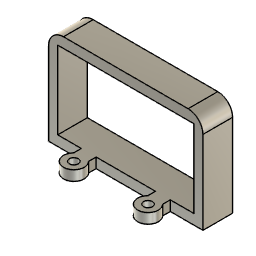
bat checker v5 (Autodesk Fusion 360 design; units mm, degrees)
Autodesk Fusion 360 part; units mm, degrees
note: some values were not read from the file. Set by a fixed rule: which sketch regions a step uses.
sketch "Sketch1" plane through (0, 0, 0) normal (0, 0, 1) x (1, 0, 0)
  line L0 (-65, 40) -> (-15, 40)
  line L1 (-15, 40) -> (-15, 50)
  line L2 (-15, 50) -> (-65, 50)
  line L3 (-65, 50) -> (-65, 40)
  dimension "d15" = 50
  constraint horizontal L0
  constraint vertical L1
  constraint horizontal L2
  constraint vertical L3
  measures "d15" distance of L0.start L0.end
extrude "Extrude4" add sketch "Sketch1" along normal blind 3
sketch "Sketch5" plane through (0, 0, 0) normal (0, 0, -1) x (1, 0, 0)
  line L0 (-65, -40) -> (-65, -50)
  line L1 (-65, -50) -> (-15, -50)
  line L2 (-15, -50) -> (-15, -40)
  line L3 (-15, -40) -> (-65, -40)
  line L4 (-65, -45) -> (-15, -45)
  line L5 (-15, -45) -> (-15, -50)
  line L6 (-15, -50) -> (-65, -50)
  line L7 (-65, -50) -> (-65, -45)
  constraint horizontal L4
  constraint vertical L5
  constraint horizontal L6
  constraint vertical L7
  constraint coincident L1.end L2.start
  constraint midpoint L0 L4.start
extrude "Extrude5" add sketch "Sketch5" along normal blind 30 contours L0 L1 L2 L4 L5 L6 L7
sketch "Sketch6" plane through (0, 50, 0) normal (0, 1, 0) x (-1, 0, 0)
  line L0 (65, -30) -> (65, 3)
  line L1 (65, 3) -> (15, 3)
  line L2 (15, 3) -> (15, -30)
  line L3 (15, -30) -> (65, -30)
  line L4 (17.55, -0.4) -> (62.45, -0.4)
  line L5 (62.45, -0.4) -> (62.45, -26.6)
  line L6 (62.45, -26.6) -> (17.55, -26.6)
  line L7 (17.55, -26.6) -> (17.55, -0.4)
  line L8 (17.55, -0.4) -> (62.45, -26.6) construction
  line L9 (62.45, -0.4) -> (17.55, -26.6) construction
  point P0 (40, -13.5)
  dimension "d24" = 44.9
  dimension "d25" = 26.2
  constraint horizontal L4
  constraint perpendicular L4 L5
  constraint parallel L4 L6
  constraint parallel L5 L7
  constraint coincident L8 P0
  constraint coincident L9 P0
  measures "d24" distance of L5.end L6.end
  measures "d25" distance of L4.end L5.end
extrude "Extrude6" cut sketch "Sketch6" against normal blind 8 contours L4 L5 L6 L7
fillet "Fillet1" radius 5 2 edges at (-65, 47.5, -30) (-15, 47.5, -30)
fillet "Fillet3" radius 2 1 edges at (-15, 40, 1.5)
sketch "Sketch7" plane through (0, 0, 0) normal (0, 0, -1) x (1, 0, 0)
  arc A0 (-15, -42) -> (-17, -40) centre (-17, -42) ccw
  line L0 (-17, -40) -> (-65, -40)
  line L1 (-65, -40) -> (-65, -45)
  line L2 (-65, -45) -> (-15, -45)
  line L3 (-15, -45) -> (-15, -42)
extrude "Extrude7" cut 1 faces at (-32.3333, 43.3333, 0) along direction (0, 0, 1) blind 10
sketch "Sketch8" plane through (0, 0, 3) normal (0, 0, 1) x (-1, 0, 0)
  line L0 (65, -45) -> (15, -45)
  line L1 (15, -45) -> (15, -50)
  line L2 (15, -50) -> (65, -50)
  line L3 (65, -50) -> (65, -45)
  line L4 (25, -50) -> (30, -50)
  line L5 (30, -50) -> (30, -40)
  line L6 (30, -40) -> (25, -40)
  line L7 (25, -40) -> (25, -50)
  line L8 (50, -50) -> (55, -50)
  line L9 (55, -50) -> (55, -40)
  line L10 (55, -40) -> (50, -40)
  line L11 (50, -40) -> (50, -50)
  circle A0 centre (27.5, -40) radius 1.5
  circle A1 centre (52.5, -40) radius 1.5
  circle A2 centre (27.5, -40) radius 3.5
  circle A3 centre (52.5, -40) radius 3.5
  dimension "d36" = 3
  dimension "d37" = 3
  dimension "d38" = 2
  dimension "d39" = 2
  constraint horizontal L4
  constraint vertical L5
  constraint horizontal L6
  constraint vertical L7
  constraint coincident L2 L4.start
  constraint horizontal L8
  constraint vertical L9
  constraint horizontal L10
  constraint vertical L11
  constraint coincident L2 L8.start
  constraint midpoint L6 A0.centre
  constraint midpoint L10 A1.centre
  measures "d36" diameter of A0
  measures "d37" diameter of A1
extrude "Extrude8" add sketch "Sketch8" against normal blind 2 contours L0 L2 L8 L9 L11 | L0 L9 L11 A3 | L9 L10 L11 A1 A3 | L9 L10 L11 A1 A3 | L0 L2 L4 L5 L7 | L0 L5 L7 A2 | L5 L6 L7 A0 A2 | L5 L6 L7 A0 A2
sketch "Sketch9" plane through (0, 0, 3) normal (0, 0, 1) x (-1, 0, 0)
  circle A0 centre (27.5, -40) radius 1.5
  line L0 (15, -50) -> (65, -50)
  line L1 (65, -50) -> (65, -45)
  line L2 (65, -45) -> (55, -45)
  line L3 (55, -45) -> (55, -42.4495)
  arc A1 (55, -42.4495) -> (50, -42.4495) centre (52.5, -40) ccw
  line L4 (50, -42.4495) -> (50, -45)
  line L5 (50, -45) -> (30, -45)
  line L6 (30, -45) -> (30, -42.4495)
  arc A2 (30, -42.4495) -> (25, -42.4495) centre (27.5, -40) ccw
  line L7 (25, -42.4495) -> (25, -45)
  line L8 (25, -45) -> (15, -45)
  line L9 (15, -45) -> (15, -50)
  circle A3 centre (52.5, -40) radius 1.5
  circle A4 centre (27.5, -40) radius 1.5
  circle A5 centre (52.5, -40) radius 1.5
  circle A6 centre (27.5, -40) radius 2
  circle A7 centre (52.5, -40) radius 2
  dimension "d42" = 4
  dimension "d43" = 4
  constraint concentric A0 A6
  constraint concentric A5 A7
  measures "d42" diameter of A6
  measures "d43" diameter of A7
extrude "Extrude9" cut sketch "Sketch9" against normal blind 5 contours A6
move_body "Move1" bodies 1 to x (-1, 0, 0) y (0, 1, 0) z (0, 0, -1) at (-130, 0, -60)
sketch "Sketch10" plane through (0, 0, -61) normal (0, 0, 1) x (-1, 0, 0)
  circle A0 centre (102.5, -40) radius 2
  line L0 (100, -45) -> (105, -45)
  line L1 (105, -45) -> (105, -42.4495)
  arc A1 (105, -42.4495) -> (100, -42.4495) centre (102.5, -40) ccw
  line L2 (100, -42.4495) -> (100, -45)
  circle A2 centre (102.5, -40) radius 1.5
  dimension "d46" = 3
  constraint concentric A0 A2
  measures "d46" diameter of A2
extrude "Extrude10" add sketch "Sketch10" against normal blind 2 contours A0
extrude "Extrude11" add 1 faces at (-115, 46.6667, -53.6667) along direction (-1, 0, 0) blind 1
extrude "Extrude12" add 1 faces at (-65, 48.3333, -44.3333) along direction (1, 0, 0) blind 2
extrude "Extrude13" add 1 faces at (-64.3333, 46.6667, -35) along direction (0, 0, 1) blind 5
extrude "Extrude14" cut 1 faces at (-63, 46.6667, -41) along direction (-1, 0, 0) blind 1
extrude "Extrude15" add 1 faces at (-115.3333, 48.3333, -35) along direction (0, 0, 1) blind 5
extrude "Extrude16" add 1 faces at (-115, 48.3333, -33.3333) along direction (1, 0, 0) blind 2
extrude "Extrude17" add 1 faces at (-113, 48.3333, -30.6667) along direction (1, 0, 0) blind 4
extrude "Extrude18" add 1 faces at (-65, 46.6667, -33.3333) along direction (-1, 0, 0) blind 2
extrude "Extrude19" add 1 faces at (-67, 46.6667, -30.6667) along direction (-1, 0, 0) blind 5
extrude "Extrude20" cut 1 faces at (-67.55, 48.3333, -50.8667) along direction (1, 0, 0) blind 0.5
extrude "Extrude21" cut 1 faces at (-112.45, 46.6667, -42.1333) along direction (-1, 0, 0) blind 0.5
extrude "Extrude22" add 1 faces at (-82.35, 50, -61.8667) along direction (0, 1, 0) blind 5
fillet "Fillet4" radius 5 1 edges at (-116, 50, -30)
fillet "Fillet5" radius 5 1 edges at (-64, 50, -30)
extrude "Extrude23" add 2 faces at (-77.5374, 43.8319, -61) (-102.5374, 43.8319, -61) along direction (0, 0, 1) blind 1.4
